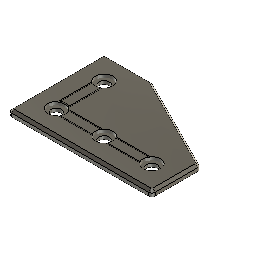
EXTRUSIONbracket (Autodesk Fusion 360 design; units mm, degrees)
Autodesk Fusion 360 part; units mm, degrees
note: some values were not read from the file. Set by a fixed rule: which face or edge a step refers to.
sketch "bracketSketch" plane through (0, 0, 0) normal (0, 0, 1) x (1, 0, 0)
  line L0 (0, 0) -> (90, 0)
  line L1 (90, 0) -> (90, 60)
  line L2 (90, 60) -> (0, 60)
  line L3 (0, 60) -> (0, 0)
  line L4 (0, 15) -> (90, 15) construction
  line L5 (15, 0) -> (15, 60) construction
  line L6 (0, 45) -> (90, 45) construction
  line L7 (75, 0) -> (75, 60) construction
  line L8 (15, 12) -> (75, 12)
  arc A0 (75, 12) -> (75, 18) centre (75, 15) ccw
  line L9 (75, 18) -> (15, 18)
  arc A1 (15, 18) -> (15, 12) centre (15, 15) ccw
  line L10 (15, 15) -> (75, 15) construction
  line L11 (18, 15) -> (18, 45)
  arc A2 (18, 45) -> (12, 45) centre (15, 45) ccw
  line L12 (12, 45) -> (12, 15)
  arc A3 (12, 15) -> (18, 15) centre (15, 15) ccw
  line L13 (15, 15) -> (15, 45) construction
  line L14 (19, 57) -> (11, 57)
  line L15 (11, 57) -> (11, 33)
  line L16 (11, 33) -> (19, 33)
  line L17 (19, 33) -> (19, 57)
  line L18 (19, 57) -> (11, 33) construction
  line L19 (11, 57) -> (19, 33) construction
  line L20 (19, 37) -> (11, 37)
  line L21 (11, 37) -> (11, 53)
  line L22 (11, 53) -> (19, 53)
  line L23 (19, 53) -> (19, 37)
  line L24 (19, 37) -> (11, 53) construction
  line L25 (11, 37) -> (19, 53) construction
  line L26 (87, 19) -> (63, 19)
  line L27 (63, 19) -> (63, 11)
  line L28 (63, 11) -> (87, 11)
  line L29 (87, 11) -> (87, 19)
  line L30 (87, 19) -> (63, 11) construction
  line L31 (63, 19) -> (87, 11) construction
  line L32 (83, 19) -> (67, 19)
  line L33 (67, 19) -> (67, 11)
  line L34 (67, 11) -> (83, 11)
  line L35 (83, 11) -> (83, 19)
  line L36 (83, 19) -> (67, 11) construction
  line L37 (67, 19) -> (83, 11) construction
  point P0 (15, 45)
  point P1 (15, 45)
  point P2 (75, 15)
  point P3 (75, 15)
  dimension "d1" = 90
  dimension "d2" = 60
  dimension "d3" = 15
  dimension "d4" = 15
  dimension "d10" = 15
  dimension "d11" = 15
  dimension "d38" = 6
  dimension "d39" = 6
  dimension "d61" = 8
  dimension "d62" = 24
  dimension "d63" = 8
  dimension "d64" = 16
  dimension "d65" = 24
  dimension "d66" = 8
  dimension "d67" = 16
  dimension "d68" = 8
  constraint horizontal L0
  constraint vertical L1
  constraint horizontal L2
  constraint vertical L3
  constraint coincident L0.start L3.end
  constraint coincident L3 L4.start
  constraint coincident L1 L4.end
  constraint perpendicular L1 L4
  constraint coincident L0 L5.start
  constraint coincident L2 L5.end
  constraint perpendicular L2 L5
  constraint coincident L3 L6.start
  constraint coincident L1 L6.end
  constraint perpendicular L1 L6
  constraint coincident L0 L7.start
  constraint coincident L2 L7.end
  constraint perpendicular L2 L7
  constraint tangent L8 A0
  constraint tangent A0 L9
  constraint parallel L8 L9
  constraint tangent L9 A1
  constraint tangent L8 A1
  constraint coincident L4 P3
  constraint coincident L7 P3
  constraint perpendicular L7 L10
  constraint coincident L5 A1.centre
  constraint tangent L11 A2
  constraint tangent A2 L12
  constraint parallel L11 L12
  constraint tangent L12 A3
  constraint tangent L11 A3
  constraint coincident L6 P1
  constraint coincident L5 P1
  constraint perpendicular L6 L13
  constraint coincident A1.centre L10.start
  constraint horizontal L14
  constraint perpendicular L14 L15
  constraint parallel L14 L16
  constraint parallel L15 L17
  constraint coincident L18 P1
  constraint coincident L19 P1
  constraint coincident P1 P0
  constraint horizontal L20
  constraint perpendicular L20 L21
  constraint parallel L20 L22
  constraint parallel L21 L23
  constraint coincident L24 P1
  constraint coincident L25 P1
  constraint horizontal L26
  constraint perpendicular L26 L27
  constraint parallel L26 L28
  constraint parallel L27 L29
  constraint coincident L30 P3
  constraint coincident L31 P3
  constraint coincident P3 P2
  constraint horizontal L32
  constraint perpendicular L32 L33
  constraint parallel L32 L34
  constraint parallel L33 L35
  constraint coincident L36 P3
  constraint coincident L37 P3
  measures "d1" distance of L0.start L0.end
  measures "d2" distance of L0.start L2.end
  measures "d3" distance of L0 L4
  measures "d4" distance of L3 L5
  measures "d10" distance of L2 L6
  measures "d11" distance of L1 L7
  measures "d38" diameter of A0
  measures "d39" diameter of A2
  measures "d61" distance of L15.end L16.end
  measures "d62" distance of L14.end L15.end
  measures "d63" distance of L21.end L22.end
  measures "d64" distance of L20.end L21.end
  measures "d65" distance of L27.end L28.end
  measures "d66" distance of L26.end L27.end
  measures "d67" distance of L33.end L34.end
  measures "d68" distance of L32.end L33.end
extrude "Extrude1" add sketch "bracketSketch" along normal blind 4 contours L0 L1 L2 L3 | L8 L9 L11 A3 L27 | L9 A1 L11 A3 | L8 L9 L27 L33 | L8 L27 L28 L33 | L9 A1 L11 L12 L16 | L8 A0 L9 L33 | L8 A0 L9 L26 L28 L32 L33 L34 L35 | L9 L26 L27 L33 | L12 L15 L16 L20 | L11 L12 L16 L20 | L11 A2 L12 L15 L17 L20 L21 L22 L23 | L11 A2 L12 L20 | L11 L16 L17 L20 | L26 L28 L29 L35 | L14 L15 L17 L22 picked at (57.333333, 44) picked at (48, 15) picked at (15.334961, 15.101936) picked at (64.333333, 16) picked at (65.666667, 11.333333) picked at (15, 28) picked at (72.333333, 16) picked at (81.330537, 14.92527) picked at (64.333333, 18.666667) picked at (11.333333, 34.333333) picked at (14, 35.666667) picked at (15.07473, 51.330537) picked at (14, 42.333333) picked at (18.666667, 34.333333) picked at (84.333333, 16.333333) picked at (13.666667, 55.666667)
sketch "Sketch3" plane through (0, 0, 4) normal (0, 0, 1) x (-1, 0, 0)
  line L0 (0, -60) -> (0, 0)
  line L1 (0, 0) -> (-90, 0)
  line L2 (-90, 0) -> (-90, -60)
  line L3 (-90, -60) -> (0, -60)
  line L4 (0, -60) -> (0, 0)
  line L5 (0, 0) -> (-90, 0)
  point P0 (-15, -15)
  dimension "d46" = 15
  dimension "d47" = 15
  measures "d46" distance of P0 L4
  measures "d47" distance of P0 L5
chamfer "Chamfer4" distance 30 distance2 60 1 edges at (90, 60, 2) measured on face at (90, 20, 1.333333)
hole "Hole1" at (15, 15, 4) direction (0, 0, -1) diameter 6.5 depth 6 tip angle 180 counterbore diameter 11 counterbore depth 2
extrude "Extrude2" cut sketch "bracketSketch" along normal blind 0.4 from surface at 3.6 contours L8 L9 L11 A3 L27 | L9 A1 L11 A3 | L8 L9 L27 L33 | L9 A1 L11 L12 L16 | L8 A0 L9 L33 | L11 L12 L16 L20 | L11 A2 L12 L20 picked at (48, 15) picked at (15.334961, 15.101936) picked at (64.333333, 16) picked at (15, 28) picked at (72.333333, 16) picked at (14, 35.666667) picked at (14, 42.333333)
chamfer "Chamfer8" distance 0.4 angle 45 6 edges at (12, 32.304886, 4) (15, 48, 4) (18, 32.304886, 4) (47.304886, 18, 4) (78, 15, 4) (47.304886, 12, 4)
extrude "Extrude4" add 8 faces at (56.536591, 12, 3.600053) (56.833333, 15, 3.6) (38.073182, 18, 3.600053) (76.165304, 12.235571, 3.600053) (12, 36.536591, 3.600053) (15, 36.833333, 3.6) (18, 36.536591, 3.600053) (12.003729, 45.149538, 3.600053) along direction (0, 0, 1) blind 0.4
chamfer "Chamfer9" distance 0.4 angle 45 2 faces at (15, 36.833333, 4) (56.833333, 15, 4)
pattern_linear "R-Pattern1" count 2 spacing 30 along (0, 1, 0) of "Hole1"
pattern_linear "R-Pattern2" count 3 spacing 30 along (1, 0, 0) of "Hole1"
extrude "Extrude6" add sketch "bracketSketch" against normal blind 2 contours L8 L9 L27 L33 | L8 L27 L28 L33 | L9 L26 L27 L33 | L26 L28 L29 L35 picked at (64.333333, 16) picked at (65.666667, 11.333333) picked at (64.333333, 18.666667) picked at (84.333333, 16.333333)
chamfer "Chamfer10" distance 0.5 angle 45 2 faces at (84.333333, 16.333333, -2) (65.666667, 13.666667, -2)
extrude "Extrude7" add sketch "bracketSketch" against normal blind 2 contours L12 L15 L16 L20 | L11 L12 L16 L20 | L11 L16 L17 L20 | L14 L15 L17 L22 picked at (11.333333, 34.333333) picked at (14, 35.666667) picked at (18.666667, 34.333333) picked at (13.666667, 55.666667)
chamfer "Chamfer11" distance 0.5 angle 45 2 faces at (16.333333, 34.333333, -2) (13.666667, 55.666667, -2)
pattern_linear "R-Pattern3" count 1 spacing 30 along (0, -1, 0) of "Extrude7", "Chamfer11"
pattern_linear "R-Pattern4" count 2 spacing 30 along (-1, 0, 0) of "Extrude6", "Chamfer10"
fillet "Fillet2" radius 2 5 edges at (90, 0, 2) (0, 60, 2) (0, 0, 2) (90, 30, 2) (30, 60, 2)
chamfer "Chamfer5" distance 0.5 angle 45 10 edges at (90, 15.381966, 0) (89.701302, 29.815394, 0) (59.658359, 45.17082, 0) (29.98737, 59.946498, 0) (15.763932, 60, 0) (0.585786, 59.414214, 0) (0, 30, 0) (0.585786, 0.585786, 0) (45, 0, 0) (89.414214, 0.585786, 0)
chamfer "Chamfer5" distance 1.5 angle 45 10 edges at (90, 15.381966, 4) (89.701302, 29.815394, 4) (59.658359, 45.17082, 4) (29.98737, 59.946498, 4) (15.763932, 60, 4) (0.585786, 59.414214, 4) (0, 30, 4) (0.585786, 0.585786, 4) (45, 0, 4) (89.414214, 0.585786, 4)
equation "d1 = ( unitsX * 30 ) * 1 mm"
equation "d2 = ( unitsY * 30 ) * 1 mm"
equation "d5 = thickness"
equation "d15 = thickness + 2 mm"
equation "d19 = unitsY"
equation "d23 = unitsX"
equation "d27 = thickness - 2 mm"
equation "d34 = ( ( unitsY - 1 ) * 30 ) * 1 mm"
equation "unitsX = 3"
equation "unitsY = 2"
equation "d40 = thickness - 0.4 mm"
equation "d48 = ( ( unitsX - 1 ) * 30 ) * 1 mm"
equation "thickness = 4 mm"
equation "d74 = unitsY - 1"
equation "d78 = unitsX - 1"
